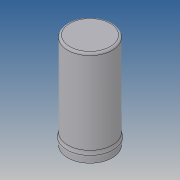
# Autodesk Inventor part: Löffelbox_oben
Saved by Autodesk Inventor 2019.4 (Build 234330000, 330)
## iProperties
Created: 2020-09-25
Part Number: Löffelbox_oben
Material: GEDA Stahl
Document SubType Name: Modeling
Designer: Admin
Mass: 193.859 g
Surface Area: 249.694 cm^2
Volume: 24.664 cm^3
Density: 7.86 g/cm^3
Appearance: GEDA Stahl A
Gewicht: 0,194 kg
G_L: 0
G_H: 0
G_B: 0
VAULT_Status: In Bearbeitung
Revision: -
Max. Breite: 0
Max. Höhe: 0
Max. Länge: 0
Max. Abmessungen: 0 x 0 x 0
Anfängl. Veröffentlichungsdatum: 2020-02-13
Volumen: 24663,956
InventorVersion: 2019.4
Author: Admin
Autodesk Inventor part; units mm, degrees
note: some values were not read from the file. Chosen so that the rebuilt part matches the saved one: edges of "Rundung2". Left out: dimensions or parameters whose unit could not be read.
ref_plane "YZ Plane" through (0, 0, 0) normal (1, 0, 0) x (0, 1, 0)
ref_plane "XZ Plane" through (0, 0, 0) normal (0, 1, 0) x (-1, 0, 0)
ref_plane "XY Plane" through (0, 0, 0) normal (0, 0, 1) x (1, 0, 0)
sketch "Skizze1" plane through (0, 0, 0) normal (0, 0, 1) x (1, 0, 0)
  circle A0 centre (0, 0) radius 19
  circle A1 centre (0, 0) radius 21
  dimension "d0" = 38
  dimension "d1" = 2
  constraints: 2 centre point, 2 coincident
  measures "d0" diameter of A0
  measures "d1" radial gap between concentric circles of A1 A0
extrude "Extrusion1" add sketch "Skizze1" along normal blind 80
sketch "Skizze2" plane through (0, 0, 80) normal (0, 0, 1) x (1, 0, 0)
  circle A0 centre (0, 0) radius 21 projected
extrude "Extrusion2" add sketch "Skizze2" along normal blind 1.8
fillet "Rundung1" radius 2 2 edges at (-21, 0, 81.8) (-19, 0, 80)
sketch "Skizze3" plane through (0, 0, 0) normal (1, 0, 0) x (0, 1, 0)
  line L0 (-21, 0) -> (21, 0) projected
  line L1 (21, 0) -> (23, -2.5) construction
  line L2 (23, -2.5) -> (21, -4) construction
  line L3 (21, -4) -> (21, -8) construction
  spline S0 degree 3 poles (21, 0) (23, -2.5) (21, -4) (21, -8) knots 1 1 1 1 2 2 2 2
  spline S1 degree 2 poles (19, 0) (21, -2.5) (19, -5) knots 0 0 0 1 1 1
  line L4 (19, -5) -> (19, -8)
  line L5 (19, -8) -> (21, -8)
  line L6 (21, 0) -> (19, 0)
  line L7 (21, 0) -> (21, 79.8) projected
  line L8 (21, 0) -> (21, 79.8) projected
  line L9 (0, -25.6969) -> (0, 97.3828) projected
  point P0 (0, 0)
  point P1 (20, -2.5)
  dimension "d7" = 2
  dimension "d8" = 2
  dimension "d9" = 8
  dimension "d10" = 1
  dimension "d11" = 2.5
  dimension "d12" = 5
  dimension "d13" = 4
  constraints: 6 end point, 2 vertical, 1 collinear, 1 horizontal alignment, 1 parallel, 1 perpendicular, 1 point on line, 1 vertical alignment, 6 other
  measures "d7" distance of L4.end L3.end
  measures "d8" distance from line of L3 L1.end
  measures "d9" distance between parallel lines of L5 L0
  measures "d10" distance from line of L4 point (20, -2.5)
  measures "d11" vertical distance of L4.start point (20, -2.5)
  measures "d12" distance of L6.end L4.start
  measures "d13" distance of L2.end L3.end
revolve "Umdrehung1" add sketch "Skizze3" angle 360 about axis through (0, 0, -10) along (0, 0, 1)
fillet "Rundung2" radius 10 1 edges at (14.8492, 14.8492, 0)
chamfer "Fase1" distance 1 angle 45 1 edges at (0, -19, -8)
equation "\"d11\" = 0.5 * d12"
equation "\"G_L\" = 0"
equation "\"G_H\" = 0"
equation "\"G_B\" = 0"
